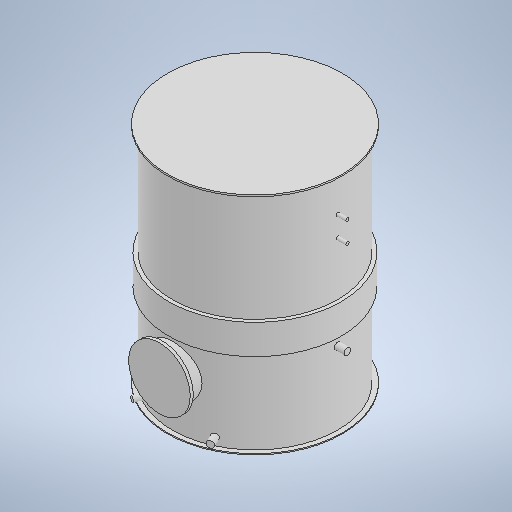
# Autodesk Inventor part: NDM-VOS dummy3
Saved by Autodesk Inventor 2025 (Build 290162010, 162A)
## iProperties
Created: 2024-09-27
Part Number: NDM-VOS dummy3
Material: Generic
Document SubType Name: Modeling
Designer: DELL
Density: 1 g/cm^3
Appearance: Default
Author: DELL
Autodesk Inventor part; units mm, degrees
ref_plane "YZ Plane" through (0, 0, 0) normal (1, 0, 0) x (0, 1, 0)
ref_plane "XY Plane" through (0, 0, 0) normal (0, 0, 1) x (1, 0, 0)
sketch "Sketch3" plane through (0, 0, 0) normal (0, 1, 0) x (-1, 0, 0)
  line L0 (0, 0) -> (0, 2190)
  line L1 (0, 2190) -> (-850, 2190)
  line L2 (-850, 2190) -> (-850, 2174)
  line L3 (-850, 2174) -> (-805, 2174)
  line L4 (-805, 2174) -> (-805, 10)
  line L5 (-805, 10) -> (-850, 10)
  line L6 (-850, 10) -> (-850, 0)
  line L7 (-850, 0) -> (0, 0)
  line L8 (-805, 1110) -> (-840, 1110)
  line L9 (-840, 1110) -> (-840, 820)
  line L10 (-840, 820) -> (-805, 820)
  dimension "d3" = 2190
  dimension "d4" = 10
  dimension "d6" = 1610
  dimension "d7" = 1700
  dimension "d8" = 16
  dimension "d9" = 290
  dimension "d10" = 810
  dimension "d11" = 1680
  constraints: 22 end point, 9 perpendicular, 2 point on line, 1 horizontal, 1 parallel, 1 vertical
  measures "d3" distance of L0.start L0.end
  measures "d4" distance of L5.end L6.end
  measures "d6" diameter of L4 L0
  measures "d7" diameter of L6 L0
  measures "d8" distance of L1.end L2.end
  measures "d9" distance of L8.end L9.end
  measures "d10" distance between parallel lines of L10 L5
  measures "d11" diameter of L9 L0
revolve "Revolution1" add sketch "Sketch3" angle 360 about axis through (0, 0, 0) along (0, 0, 1)
sketch "Sketch4" plane through (0, 0, 0) normal (0, 1, 0) x (-1, 0, 0)
  circle A0 centre (0, 510) radius 250
  line L0 (805, 10) -> (-805, 10) projected
  point P0 (0, 0)
  point P1 (0, 10)
  dimension "d13" = 500
  dimension "d14" = 500
  constraints: 1 centre point, 1 midpoint, 1 vertical alignment
  measures "d13" diameter of A0
  measures "d14" distance from line of L0 A0.centre
extrude "Extrusion2" add sketch "Sketch4" against normal blind 900
sketch "Sketch5" plane through (0, -900, 510) normal (0, -1, 0) x (1, 0, 0)
  circle A0 centre (0, 0) radius 250 construction
  circle A1 centre (0, 0) radius 300
  point P0 (0, -510)
  dimension "d17" = 600
  constraints: 1 centre point, 1 coincident
  measures "d17" diameter of A1
extrude "Extrusion3" add sketch "Sketch5" along normal blind 30
sketch "Sketch6" plane through (0, 0, 0) normal (1, 0, 0) x (0, 1, 0)
  circle A0 centre (0, 720) radius 32.5
  circle A1 centre (0, 1830) radius 16
  circle A2 centre (0, 1630) radius 16
  line L0 (805, 10) -> (-805, 10) projected
  point P0 (0, 0)
  dimension "d20" = 710
  dimension "d21" = 1820
  dimension "d22" = 1620
  dimension "d23" = 32
  dimension "d24" = 65
  constraints: 3 centre point, 3 vertical alignment, 1 equal radius
  measures "d20" distance from line of A0.centre L0
  measures "d21" distance from line of A1.centre L0
  measures "d22" distance from line of A2.centre L0
  measures "d23" diameter of A2
  measures "d24" diameter of A0
extrude "Extrusion4" add sketch "Sketch6" along normal blind 900
sketch "Sketch7" plane through (0, 0, 0) normal (0, 1, 0) x (-1, 0, 0)
  circle A0 centre (0, 300) radius 16
  circle A1 centre (0, 720) radius 32.5
  circle A2 centre (0, 1370) radius 32.5
  line L0 (805, 10) -> (-805, 10) projected
  point P0 (0, 0)
  point P1 (0, 10)
  dimension "d27" = 300
  dimension "d28" = 710
  dimension "d29" = 1360
  dimension "d30" = 65
  dimension "d31" = 32
  constraints: 3 centre point, 3 vertical alignment, 1 equal radius, 1 midpoint
  measures "d27" distance of point (0, 0) A0.centre
  measures "d28" distance from line of L0 A1.centre
  measures "d29" distance from line of L0 A2.centre
  measures "d30" diameter of A2
  measures "d31" diameter of A0
extrude "Extrusion5" add sketch "Sketch7" along normal blind 900
ref_plane "Work Plane1" through (0, 0, 0) normal (-0.4226183, 0.9063078, 0) x (0, 0, 1)
sketch "Sketch8" plane through (0, 0, 0) normal (-0.4226183, 0.9063078, 0) x (0, 0, 1)
  circle A0 centre (85, 0) radius 32.5
  point P0 (0, 0)
  dimension "d35" = 65
  dimension "d36" = 85
  constraints: 1 centre point, 1 horizontal alignment
  measures "d35" diameter of A0
  measures "d36" distance of A0.centre point (0, 0)
extrude "Extrusion6" add sketch "Sketch8" against normal blind 900
ref_plane "Work Plane2" through (0, 0, 0) normal (0.4226183, 0.9063078, 0) x (0, 0, 1)
sketch "Sketch9" plane through (0, 0, 0) normal (0.4226183, 0.9063078, 0) x (0, 0, 1)
  circle A0 centre (85, 0) radius 25
  point P0 (0, 0)
  dimension "d40" = 50
  dimension "d41" = 85
  constraints: 1 centre point, 1 horizontal alignment
  measures "d40" diameter of A0
  measures "d41" distance of point (0, 0) A0.centre
extrude "Extrusion7" add sketch "Sketch9" against normal blind 900
body "Solid2"
